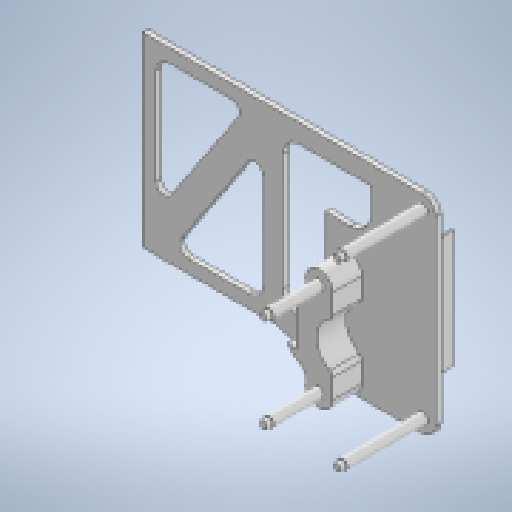
# Autodesk Inventor part: CaseBase
Saved by Autodesk Inventor 2025.2 (Build 292293000, 293)
## iProperties
Created: 2026-02-21
Part Number: CaseBase
Material: 一般
Document SubType Name: Modeling
Designer: naka6
Density: 1 g/cm^3
Appearance: 既定
Author: naka6
Autodesk Inventor part; units mm, degrees
ref_plane "YZ Plane" through (0, 0, 0) normal (1, 0, 0) x (0, 1, 0)
ref_plane "XZ Plane" through (0, 0, 0) normal (0, 1, 0) x (-1, 0, 0)
ref_plane "XY Plane" through (0, 0, 0) normal (0, 0, 1) x (1, 0, 0)
sketch "スケッチ1" plane through (0, 0, 0) normal (0, 0, 1) x (1, 0, 0)
  circle A0 centre (0, 0) radius 1.5 projected
  line L0 (5, 28) -> (5, 19) projected
  arc A1 (-3, 11) -> (5, 19) centre (-3, 19) ccw projected
  line L1 (-3, 11) -> (-12, 11) projected
  line L2 (-12, 11) -> (-12, -28) projected
  line L3 (-12, -28) -> (22, -28) projected
  arc A2 (22, -28) -> (28, -22) centre (22, -22) ccw projected
  line L4 (28, -22) -> (28, 22) projected
  arc A3 (28, 22) -> (22, 28) centre (22, 22) ccw projected
  line L5 (22, 28) -> (5, 28) projected
  line L6 (29.2, 50) -> (-80.8, 50)
  line L7 (-80.8, 50) -> (-80.8, -50)
  line L8 (-80.8, -50) -> (29.2, -50)
  line L9 (29.2, -50) -> (29.2, 50)
  line L10 (29.2, 0) -> (-80.8, 0)
  line L11 (22, -28) -> (-22, -28) projected
  arc A4 (-28, -22) -> (-22, -28) centre (-22, -22) ccw projected
  line L12 (-28, -22) -> (-28, 22) projected
  arc A5 (-22, 28) -> (-28, 22) centre (-22, 22) ccw projected
  line L13 (-22, 28) -> (22, 28) projected
  arc A6 (28, 22) -> (22, 28) centre (22, 22) ccw projected
  line L14 (28, 22) -> (28, -22) projected
  arc A7 (22, -28) -> (28, -22) centre (22, -22) ccw projected
  circle A8 centre (0, 0) radius 80 projected
  line L15 (22, 28.2) -> (-22, 28.2)
  arc A9 (-22, 28.2) -> (-28.2, 22) centre (-22, 22) ccw
  line L16 (-28.2, 22) -> (-28.2, -22)
  arc A10 (-28.2, -22) -> (-22, -28.2) centre (-22, -22) ccw
  line L17 (-22, -28.2) -> (22, -28.2)
  arc A11 (28.2, 22) -> (22, 28.2) centre (22, 22) ccw
  line L18 (28.2, -22) -> (28.2, 22)
  arc A12 (22, -28.2) -> (28.2, -22) centre (22, -22) ccw
  line L19 (29.2, -22) -> (29.2, 22)
  arc A13 (29.2, 22) -> (22, 29.2) centre (22, 22) ccw
  line L20 (22, 29.2) -> (-22, 29.2)
  arc A14 (-22, 29.2) -> (-29.2, 22) centre (-22, 22) ccw
  line L21 (-29.2, 22) -> (-29.2, -22)
  arc A15 (-29.2, -22) -> (-22, -29.2) centre (-22, -22) ccw
  line L22 (-22, -29.2) -> (22, -29.2)
  arc A16 (22, -29.2) -> (29.2, -22) centre (22, -22) ccw
  line L23 (-12, 11) -> (-12, 28) projected
  point P0 (0, 0)
  point P1 (29.2, 0)
  dimension "d0" = 110
  dimension "d1" = 100
  dimension "d2" = 0.2
  dimension "d3" = 0.2
  dimension "d4" = 0.2
  dimension "d5" = 0.2
  dimension "d6" = 1
  dimension "d7" = 1
  dimension "d8" = 1
  dimension "d9" = 1
  constraints: 26 end point, 16 point on circle, 8 centre point, 4 midpoint, 4 parallel, 1 horizontal, 1 perpendicular, 1 point on line, 8 other
  measures "d0" distance of L8.end L7.end
  measures "d1" distance of L8.end L6.start
  measures "d2" distance between parallel lines of L13 L15
  measures "d3" radial gap between concentric circles of A3 A11
  measures "d4" distance between parallel lines of L4 L18
  measures "d5" radial gap between concentric circles of A2 A12
  measures "d6" distance between parallel lines of L18 L19
  measures "d7" radial gap between concentric circles of A11 A13
  measures "d8" distance between parallel lines of L15 L20
  measures "d9" radial gap between concentric circles of A12 A16
extrude "押し出し1" add sketch "スケッチ1" along normal blind 2 contours L10 A0 | L10 L4 A2 L3 L2 A0 | A0 L10 L2 L1 A1 L0 L5 A3 L4 | A0 L10 | L10 L18 A12 L17 A10 L16 L12 A4 L11 L3 A2 L4 | L4 A3 L5 L13 A5 L12 L10 L16 A9 L15 A11 L18 | L18 A11 L15 A9 L16 L10 L21 A14 L20 A13 L9 | L10 L9 A16 L22 A15 L21 L16 A10 L17 A12 L18 | L23 L13 L0 A1 L1 | L9 L8 A8 L10 L21 A15 L22 A16 | A13 L20 A14 L21 L10 A8 L6 L9 | A8 L8 L7 L10 | L10 L7 L6 A8
sketch "スケッチ2" plane through (0, 0, 0) normal (0, 0, -1) x (-1, 0, 0)
  line L0 (-22, -28) -> (22, -28) projected
  arc A0 (22, -28) -> (28, -22) centre (22, -22) ccw projected
  line L1 (28, -22) -> (28, 22) projected
  arc A1 (28, 22) -> (22, 28) centre (22, 22) ccw projected
  line L2 (22, 28) -> (-22, 28) projected
  arc A2 (-22, 28) -> (-28, 22) centre (-22, 22) ccw projected
  line L3 (-28, 22) -> (-28, -22) projected
  arc A3 (-28, -22) -> (-22, -28) centre (-22, -22) ccw projected
  circle A4 centre (0, 0) radius 80 projected
  line L4 (12, 11) -> (12, -28) projected
  line L5 (12, 11) -> (12, 28) projected
  line L6 (22, -28.2) -> (-22, -28.2)
  arc A5 (-28.2, -22) -> (-22, -28.2) centre (-22, -22) ccw
  line L7 (-28.2, -22) -> (-28.2, 22)
  arc A6 (-22, 28.2) -> (-28.2, 22) centre (-22, 22) ccw
  line L8 (-22, 28.2) -> (22, 28.2)
  arc A7 (28.2, 22) -> (22, 28.2) centre (22, 22) ccw
  line L9 (28.2, 22) -> (28.2, -22)
  arc A8 (22, -28.2) -> (28.2, -22) centre (22, -22) ccw
  line L10 (22, -29) -> (-22, -29)
  arc A9 (-29, -22) -> (-22, -29) centre (-22, -22) ccw
  line L11 (-29, -22) -> (-29, 22)
  arc A10 (-22, 29) -> (-29, 22) centre (-22, 22) ccw
  line L12 (-22, 29) -> (22, 29)
  arc A11 (29, 22) -> (22, 29) centre (22, 22) ccw
  line L13 (29, 22) -> (29, -22)
  arc A12 (22, -29) -> (29, -22) centre (22, -22) ccw
  line L14 (12, -28) -> (12, -29)
  line L15 (12, 28) -> (12, 29)
  line L16 (-28.2, -22) -> (-29, -22)
  line L17 (-22, -28.2) -> (-22, -29)
  line L18 (-28.2, 22) -> (-29, 22)
  line L19 (-22, 28.2) -> (-22, 29)
  point P0 (0, 0)
  point P1 (12, 28.2)
  point P2 (12, -28.2)
  dimension "d12" = 0.2
  dimension "d13" = 1
  constraints: 28 end point, 16 point on circle, 8 centre point, 4 perpendicular, 4 point on line, 14 other
  measures "d12" distance between parallel lines of L0 L6
  measures "d13" distance between parallel lines of L0 L10
extrude "押し出し2" add sketch "スケッチ2" along normal blind 5 contours L14 L10 L17 L6 | L8 L19 L12 L15 | L16 L11 L18 L7
sketch "スケッチ3" plane through (0, 0, 2) normal (0, 0, 1) x (1, 0, 0)
  line L0 (-3, 11) -> (-12, 11) projected
  arc A0 (-3, 11) -> (5, 19) centre (-3, 19) ccw projected
  line L1 (5, 28) -> (5, 19) projected
  line L2 (-12, 28.2) -> (22, 28.2) projected
  line L3 (-12, 11) -> (-12, 28) projected
  line L4 (5, 28) -> (5, 28.2)
  line L5 (-12, 28.2) -> (-12, 28)
  line L6 (5, 28) -> (-12, 28)
  point P0 (0, 0)
  constraints: 6 end point, 1 midpoint, 1 parallel, 1 vertical
extrude "押し出し3" cut sketch "スケッチ3" against normal blind 5 contours L0 L3 L6 L1 A0
sketch "スケッチ4" plane through (0, 0, 2) normal (0, 0, 1) x (1, 0, 0)
  circle A0 centre (-3.5, 19.5) radius 7 projected
  circle A1 centre (-3.5, 19.5) radius 12.5
  circle A2 centre (20.2479, 11.6875) radius 12.5
  line L0 (-3.5, 19.5) -> (-3.5, -20.5)
  line L1 (-3.5, -20.5) -> (20.2479, 11.6875)
  line L2 (-3.5, -20.5) -> (27.7695, 4.4443)
  circle A3 centre (27.7695, 4.4443) radius 12.5
  line L3 (-3.5, -3) -> (-3.5, -38)
  circle A4 centre (-3.5, -38) radius 5
  circle A5 centre (-3.5, -3) radius 5
  circle A6 centre (-3.5, -20.5) radius 14 projected
  line L4 (22, -28) -> (-22, -28) projected
  arc A7 (-28, -22) -> (-22, -28) centre (-22, -22) ccw projected
  line L5 (-28, -22) -> (-28, 22) projected
  arc A8 (-22, 28) -> (-28, 22) centre (-22, 22) ccw projected
  line L6 (-22, 28) -> (22, 28) projected
  arc A9 (28, 22) -> (22, 28) centre (22, 22) ccw projected
  line L7 (28, 22) -> (28, -22) projected
  arc A10 (22, -28) -> (28, -22) centre (22, -22) ccw projected
  circle A11 centre (0, 0) radius 80 projected
  line L8 (3.8, -22.3439) -> (3.8, -18.6561) projected
  arc A12 (6.2, -18.6561) -> (3.8, -18.6561) centre (5, -20.5) ccw projected
  line L9 (6.2, -18.6561) -> (6.2, -22.3439) projected
  arc A13 (3.8, -22.3439) -> (6.2, -22.3439) centre (5, -20.5) ccw projected
  line L10 (1.5, -3) -> (1.5, -38)
  line L11 (-12, 11) -> (-12, -28) projected
  circle A14 centre (-12, -4.9507) radius 3.721
  circle A15 centre (-11.9886, -36.0442) radius 3.711
  circle A16 centre (5, -20.5) radius 4.5 projected
  circle A17 centre (5, -20.5) radius 9.5
  point P0 (0, 0)
  point P1 (-8.3733, -4.1184)
  point P2 (-10.2152, -8.2156)
  point P3 (-12, -9.3757)
  point P4 (-15.3216, -28)
  point P5 (-10.21, -32.7872)
  point P6 (-8.3724, -36.8774)
  point P7 (1.5, -29.3318)
  point P8 (1.5, -11.6682)
  dimension "d26" = 10
  dimension "d27" = 10
  dimension "d18" = 25
  dimension "d19" = 25
  dimension "d20" = 40
  dimension "d21" = 40
  dimension "d22" = 40
  dimension "d23" = 15
  dimension "d24" = 25
  dimension "d25" = 35
  dimension "d34" = 7.422
  dimension "d35" = 5
  constraints: 10 end point, 6 centre point, 5 coincident, 3 vertical, 2 tangent, 1 collinear, 1 equal radius, 1 midpoint, 1 point on line, 8 other
  measures "d18" diameter of A1
  measures "d19" diameter of A2
  measures "d20" distance of L0.start L0.end
  measures "d21" distance of L0.end L1.end
  measures "d22" distance of L0.end L2.end
  measures "d23" angle of L2 L1
  measures "d24" diameter of A3
  measures "d25" distance of L3.start L3.end
  measures "d34" diameter of A15
  measures "d35" radial gap between concentric circles of A16 A17
extrude "押し出し4" add sketch "スケッチ4" along normal blind 11 contours A5 A6 L0 | L0 A6 A5 | L10 A6 A5 | A5 A6 A14 | L10 A17 L0 A5 A6 | A6 A5 L0 | L0 A5 A6 | A5 L0 A17 L3 L4 L11 A6 | L4 L3 A4 A6 | A17 L4 L3 | A6 A4 A15 | L4 A17 L10 A6 A4 L3 | A6 A4 | A4 L3 A6 | A4 A6 L3 | L10 A4 A6
sketch "スケッチ5" plane through (-3.5, -3, 13) normal (0, 0, 1) x (-0.9936458, -0.1125523, 0)
  arc A0 (8.6544, 33.1138) -> (-1.0289, 35.3404) centre (3.9393, 34.7776) ccw projected
  arc A1 (-4.9682, 0.5628) -> (4.9682, 0.5628) centre (0, 0) ccw projected
  circle A2 centre (3.9393, 34.7776) radius 1.9
  circle A3 centre (0, 0) radius 1.9
  point P0 (-3.8154, -2.587)
  dimension "d30" = 3.8
  dimension "d31" = 3.8
  constraints: 2 centre point, 2 coincident
  measures "d30" diameter of A2
  measures "d31" diameter of A3
extrude "押し出し5" add sketch "スケッチ5" along normal blind 19
fillet "フィレット1" radius 2 2 edges at (1.5, -11.6682, 7.5) (1.5, -29.3318, 7.5)
sketch "スケッチ6" plane through (0, 0, 2) normal (0, 0, 1) x (1, 0, 0)
  line L0 (-80.8, -35) -> (-30.8, -35)
  line L1 (-30.8, -35) -> (-30.8, 35)
  line L2 (-30.8, 35) -> (-80.8, 35)
  line L3 (-80.8, 35) -> (-80.8, -35)
  line L4 (-80.8, -35) -> (-30.8, 35) construction
  line L5 (-30.8, -35) -> (-80.8, 35) construction
  line L6 (-80.8, 50) -> (-80.8, -50) projected
  line L7 (-80.8, 0) -> (-37.8752, 0)
  line L8 (29.2, 50) -> (-80.8, 50) projected
  line L9 (29.2, 50) -> (-80.8, 50)
  line L10 (-80.8, 50) -> (-80.8, 35)
  line L11 (-80.8, 35) -> (29.2, 35)
  line L12 (29.2, 35) -> (29.2, 50)
  line L13 (-80.8, -50) -> (29.2, -50) projected
  line L14 (-80.8, -50) -> (19.0064, -50)
  line L15 (-12.8, -35) -> (-80.8, -35)
  line L16 (-80.8, -35) -> (-80.8, -50)
  line L17 (-30.8, -35) -> (19.0064, -50)
  arc A0 (-8.3724, -36.8774) -> (1.5, -38) centre (-3.5, -38) ccw projected
  line L18 (-3.5, -43) -> (29.2, -43)
  line L19 (29.2, -50) -> (29.2, 50) projected
  line L20 (-12, -29) -> (22, -29) projected
  point P0 (0, 0)
  point P1 (-55.8, 0)
  point P2 (19.0064, -50)
  point P3 (-4.9419, -42.7876)
  dimension "d37" = 50
  dimension "d38" = 70
  constraints: 32 end point, 5 horizontal, 5 parallel, 3 midpoint, 3 point on line, 2 perpendicular, 2 tangent, 1 point on circle
  measures "d37" distance of L2.end L1.end
  measures "d38" distance of L0.end L1.end
extrude "押し出し6" cut sketch "スケッチ6" against normal blind 5 contours L0 L17 L13 L6 | L2 L6 L8 L12 L11 | A0 L18 L19 L13 L17
sketch "スケッチ7" plane through (0, 0, 2) normal (0, 0, 1) x (1, 0, 0)
  circle A0 centre (-3.5, -38) radius 1.9 projected
  line L0 (-30.8, -35) -> (-4.9419, -42.7876) projected
  line L1 (29.2, -43) -> (29.2, 35) projected
  line L2 (29.2, 35) -> (-80.8, 35) projected
  line L3 (-80.8, 35) -> (-80.8, -35) projected
  line L4 (-80.8, -35) -> (-30.8, -35) projected
  arc A1 (-15.3216, -28) -> (-10.21, -32.7872) centre (-3.5, -20.5) ccw projected
  line L5 (-15.3216, -28) -> (-22, -28) projected
  arc A2 (-28, -22) -> (-22, -28) centre (-22, -22) ccw projected
  line L6 (-28, -22) -> (-28, 22) projected
  arc A3 (-22, 28) -> (-28, 22) centre (-22, 22) ccw projected
  line L7 (-22, 28) -> (5, 28) projected
  line L8 (5, 28) -> (5, 19) projected
  arc A4 (-3, 11) -> (5, 19) centre (-3, 19) ccw projected
  line L9 (-3, 11) -> (-12, 11) projected
  line L10 (-12, 11) -> (-12, -9.3757) projected
  arc A5 (-10.2152, -8.2156) -> (-12, -9.3757) centre (-3.5, -20.5) ccw projected
  arc A6 (-10.2152, -8.2156) -> (-8.3733, -4.1184) centre (-12, -4.9507) ccw projected
  arc A7 (1.5, -3) -> (-8.3733, -4.1184) centre (-3.5, -3) ccw projected
  line L11 (1.5, -3) -> (1.5, -10.4005) projected
  arc A8 (0.4565, -12.1569) -> (1.5, -10.4005) centre (-0.5, -10.4005) ccw projected
  arc A9 (0.4565, -12.1569) -> (0.4565, -28.8431) centre (5, -20.5) ccw projected
  arc A10 (1.5, -30.5995) -> (0.4565, -28.8431) centre (-0.5, -30.5995) ccw projected
  line L12 (1.5, -30.5995) -> (1.5, -38) projected
  arc A11 (-3.5, -43) -> (1.5, -38) centre (-3.5, -38) ccw projected
  arc A12 (-8.3724, -36.8774) -> (-10.21, -32.7872) centre (-11.9886, -36.0442) ccw projected
  circle A13 centre (24.2, -38) radius 1.9
  circle A14 centre (24.2, 30) radius 1.9
  arc A15 (-8.3724, -36.8774) -> (-4.9419, -42.7876) centre (-3.5, -38) ccw projected
  line L13 (-3.5, -43) -> (29.2, -43) projected
  point P0 (0, 0)
  dimension "d42" = 3.8
  dimension "d43" = 5
  dimension "d45" = 3.8
  dimension "d46" = 5
  dimension "d47" = 5
  dimension "d48" = 5
  constraints: 2 centre point
  measures "d42" diameter of A13
  measures "d43" distance from line of L1 A13.centre
  measures "d45" diameter of A14
  measures "d46" distance from line of L1 A14.centre
  measures "d47" distance from line of L2 A14.centre
  measures "d48" distance from line of L13 A13.centre
extrude "押し出し7" add sketch "スケッチ7" along normal blind 30 contours A13 | A14
fillet "フィレット2" radius 5 2 edges at (29.2, -43, 1) (29.2, 35, 1)
sketch "スケッチ8" plane through (0, 0, 2) normal (0, 0, 1) x (1, 0, 0)
  arc A0 (29.2, 30) -> (24.2, 35) centre (24.2, 30) ccw projected
  line L0 (24.2, 35) -> (-80.8, 35) projected
  line L1 (-80.8, 35) -> (-80.8, -35) projected
  line L2 (-80.8, -35) -> (-30.8, -35) projected
  line L3 (-30.8, -35) -> (-4.9419, -42.7876) projected
  arc A1 (-8.3724, -36.8774) -> (-4.9419, -42.7876) centre (-3.5, -38) ccw projected
  arc A2 (-8.3724, -36.8774) -> (-10.21, -32.7872) centre (-11.9886, -36.0442) ccw projected
  arc A3 (-15.3216, -28) -> (-10.21, -32.7872) centre (-3.5, -20.5) ccw projected
  line L4 (-15.3216, -28) -> (-22, -28) projected
  arc A4 (-28, -22) -> (-22, -28) centre (-22, -22) ccw projected
  line L5 (-28, -22) -> (-28, 22) projected
  arc A5 (-22, 28) -> (-28, 22) centre (-22, 22) ccw projected
  line L6 (-22, 28) -> (5, 28) projected
  line L7 (5, 28) -> (5, 19) projected
  arc A6 (-3, 11) -> (5, 19) centre (-3, 19) ccw projected
  line L8 (-3, 11) -> (-12, 11) projected
  line L9 (-12, 11) -> (-12, -9.3757) projected
  arc A7 (-10.2152, -8.2156) -> (-12, -9.3757) centre (-3.5, -20.5) ccw projected
  arc A8 (-10.2152, -8.2156) -> (-8.3733, -4.1184) centre (-12, -4.9507) ccw projected
  arc A9 (1.5, -3) -> (-8.3733, -4.1184) centre (-3.5, -3) ccw projected
  line L10 (1.5, -3) -> (1.5, -10.4005) projected
  arc A10 (0.4565, -12.1569) -> (1.5, -10.4005) centre (-0.5, -10.4005) ccw projected
  arc A11 (0.4565, -12.1569) -> (0.4565, -28.8431) centre (5, -20.5) ccw projected
  arc A12 (1.5, -30.5995) -> (0.4565, -28.8431) centre (-0.5, -30.5995) ccw projected
  line L11 (1.5, -30.5995) -> (1.5, -38) projected
  arc A13 (-3.5, -43) -> (1.5, -38) centre (-3.5, -38) ccw projected
  line L12 (-3.5, -43) -> (24.2, -43) projected
  arc A14 (24.2, -43) -> (29.2, -38) centre (24.2, -38) ccw projected
  line L13 (29.2, -38) -> (29.2, 30) projected
  circle A15 centre (24.2, -38) radius 1.9 projected
  circle A16 centre (24.2, 30) radius 1.9 projected
  line L14 (-80.8, -35) -> (-30.8, -35)
  line L15 (-30.8, -35) -> (-30.8, 35)
  line L16 (-30.8, 35) -> (-80.8, 35)
  line L17 (-80.8, 35) -> (-80.8, -35)
  line L18 (-35.8, 30) -> (-35.8, -30)
  line L19 (-35.8, -30) -> (-75.8, -30)
  line L20 (-75.8, -30) -> (-75.8, 30)
  line L21 (-75.8, 30) -> (-35.8, 30)
  line L22 (-30.8, 28.4861) -> (-73.1241, -35)
  line L23 (-35.8, 30) -> (-75.8, -30)
  line L24 (-38.4759, 35) -> (-80.8, -28.4861)
  point P0 (0, 0)
  point P1 (-75.8, -20.9861)
  point P2 (-41.8093, 30)
  point P3 (-35.8, 20.9861)
  point P4 (-69.7907, -30)
  dimension "d52" = 50
  dimension "d53" = 5
  dimension "d54" = 5
  dimension "d55" = 5
  constraints: 22 end point, 7 point on line, 6 parallel, 2 perpendicular, 1 horizontal, 3 other
  measures "d52" distance of L16.end L15.end
  measures "d53" distance between parallel lines of L15 L18
  measures "d54" distance between parallel lines of L22 L23
  measures "d55" distance between parallel lines of L24 L23
extrude "押し出し8" cut sketch "スケッチ8" against normal through all contours L24 L20 L21 | L18 L19 L22
fillet "フィレット3" radius 5 2 edges at (-35.8, -30, 1) (-75.8, 30, 1)
fillet "フィレット4" radius 3 4 edges at (-41.8093, 30, 1) (-35.8, 20.9861, 1) (-75.8, -20.9861, 1) (-69.7907, -30, 1)
sketch "スケッチ9" plane through (-3.5, -38, 32) normal (0, 0, 1) x (1, 0, 0)
  circle A0 centre (0, 0) radius 1.9 projected
  circle A1 centre (27.7, 0) radius 1.9 projected
  circle A2 centre (27.7, 68) radius 1.9 projected
  circle A3 centre (0, 35) radius 1.9 projected
  circle A4 centre (27.7, 68) radius 1.4
  circle A5 centre (0, 35) radius 1.4
  circle A6 centre (0, 0) radius 1.4
  circle A7 centre (27.7, 0) radius 1.4
  point P0 (3.5, 38)
  dimension "d60" = 2.8
  dimension "d61" = 2.8
  dimension "d62" = 2.8
  dimension "d63" = 2.8
  constraints: 4 centre point, 4 coincident
  measures "d60" diameter of A4
  measures "d61" diameter of A5
  measures "d62" diameter of A6
  measures "d63" diameter of A7
extrude "押し出し9" add sketch "スケッチ9" along normal blind 2 contours A4 | A5 | A6 | A7
